Autodesk Inventor part; units mm, degrees
(part 10 of 18)
  ellipse E459 centre (-107.4, -28.6975) end of major axis (-107.4136, -28.887) minor radius 0.0836 (-107.3988, -28.8851) -> (-107.3155, -28.6702) ccw
  ellipse E460 centre (-107.3023, -23.1571) end of major axis (-107.2887, -22.9676) minor radius 0.0836 (-107.2177, -23.1298) -> (-107.2887, -22.9676) ccw
  ellipse E461 centre (-107.2657, -28.7071) end of major axis (-107.2793, -28.8966) minor radius 0.0836 (-107.2644, -28.8947) -> (-107.1812, -28.6798) ccw
  line L614 (-107.423, -22.958) -> (-107.2887, -22.9676)
  line L615 (-107.9988, -29.2688) -> (-108.1215, -29.26)
  line L616 (-108.1883, -29.2815) -> (-107.9671, -29.2974)
  ellipse E462 centre (-108.0103, -29.224) end of major axis (-108.2603, -29.2257) minor radius 0.0393 (-108.2342, -29.208) -> (-108.1215, -29.26) ccw
  ellipse E463 centre (-108.0103, -29.224) end of major axis (-107.6103, -29.2214) minor radius 0.0629 (-108.3653, -29.2553) -> (-108.1883, -29.2815) ccw
  line L617 (-87.4369, -24.724) -> (-87.3368, -24.7245)
  line L618 (-87.4451, -24.7415) -> (-87.4745, -24.7414)
  line L619 (-87.3116, -26.9591) -> (-87.5116, -24.9123)
  ellipse E464 centre (-87.2873, -23.1457) end of major axis (-87.3119, -22.9573) minor radius 0.0925 (-87.2875, -22.9605) -> (-87.3058, -22.9569) ccw
  ellipse E465 centre (-86.8717, -28.7468) end of major axis (-86.8472, -28.9352) minor radius 0.0925 (-86.8533, -28.9355) -> (-86.8472, -28.9352) ccw
  line L620 (-86.8467, -28.9351) -> (-86.8472, -28.9352)
  line L621 (-87.3058, -22.9569) -> (-87.3591, -22.9566)
  line L622 (-87.2928, -28.9157) -> (-86.9898, -28.9172)
  line L623 (-87.4747, -28.9323) -> (-87.092, -28.9343)
  line L624 (-86.8543, -28.9355) -> (-86.8533, -28.9355)
  ellipse E466 centre (-87.2185, -26.9596) end of major axis (-87.194, -27.148) minor radius 0.0925 (-87.3116, -26.9591) -> (-87.2495, -27.1225) ccw
  ellipse E467 centre (-87.4185, -24.9128) end of major axis (-87.443, -24.7244) minor radius 0.0925 (-87.4369, -24.724) -> (-87.5116, -24.9123) ccw
  line L625 (-106.3707, -22.9587) -> (-106.6076, -22.9637)
  line L626 (-106.9403, -28.9202) -> (-106.6983, -28.9152)
  line L627 (-106.8323, -28.9376) -> (-106.5774, -28.9323)
  line L628 (-106.6653, -24.7299) -> (-106.5258, -24.727)
  line L629 (-106.4991, -25.3055) -> (-106.6609, -26.9609)
  line L630 (-106.4907, -24.7459) -> (-106.5311, -24.7468)
  ellipse E468 centre (-106.5443, -24.9158) end of major axis (-106.5206, -24.7273) minor radius 0.0827 (-106.4591, -24.859) -> (-106.5258, -24.727) ccw
  ellipse E469 centre (-106.7442, -26.9627) end of major axis (-106.7205, -26.7741) minor radius 0.0827 (-106.7228, -27.13) -> (-106.6609, -26.9609) ccw
  ellipse E470 centre (-106.2503, -23.0086) end of major axis (-106.6484, -22.9697) minor radius 0.023 (-106.6076, -22.9637) -> (-106.6484, -22.9697) ccw
  line L631 (-106.6484, -22.9697) -> (-106.6497, -22.983)
  line L632 (-85.8205, -29.2346) -> (-85.9837, -29.2482)
  line L633 (-85.9794, -29.275) -> (-85.746, -29.2556)
  ellipse E471 centre (-85.8192, -29.047) end of major axis (-85.8707, -29.2299) minor radius 0.1628 (-85.8205, -29.2346) -> (-85.7328, -29.1988) ccw
  ellipse E472 centre (-85.7448, -29.0679) end of major axis (-85.7963, -29.2508) minor radius 0.1628 (-85.746, -29.2556) -> (-85.6862, -29.2378) ccw
  line L634 (-86.5987, -24.7323) -> (-86.4197, -24.7827)
  line L635 (-86.2178, -25.0275) -> (-86.2312, -27.0619)
  ellipse E473 centre (-86.9459, -24.7613) end of major axis (-86.5459, -24.764) minor radius 0.0629 (-86.5987, -24.7323) -> (-87.1444, -24.7054) ccw
  line L636 (-87.3451, -24.7222) -> (-87.1444, -24.7054)
  line L637 (-87.07, -24.7264) -> (-87.4891, -24.7614)
  ellipse E474 centre (-86.9459, -24.7613) end of major axis (-87.1959, -24.7597) minor radius 0.0393 (-86.7289, -24.7432) -> (-87.07, -24.7264) ccw
  line L638 (-86.5673, -24.7887) -> (-86.7289, -24.7432)
  line L639 (-87.1603, -27.115) -> (-87.2752, -27.1246)
  ellipse E475 centre (-86.9618, -27.1709) end of major axis (-87.3618, -27.1683) minor radius 0.0629 (-86.6549, -27.1325) -> (-87.1603, -27.115) ccw
  line L640 (-86.3614, -27.0727) -> (-86.3584, -26.6213)
  line L641 (-86.3511, -25.5132) -> (-86.348, -25.0384)
  ellipse E476 centre (-86.3121, -25.001) end of major axis (-86.3279, -24.8117) minor radius 0.0933 (-86.2178, -25.0275) -> (-86.2257, -24.9475) ccw
  ellipse E477 centre (-86.3255, -27.0353) end of major axis (-86.3413, -26.846) minor radius 0.0933 (-86.2481, -27.1626) -> (-86.2312, -27.0619) ccw
  ellipse E478 centre (-86.4423, -25.0119) end of major axis (-86.4265, -25.2012) minor radius 0.0933 (-86.348, -25.0384) -> (-86.3522, -24.9791) ccw
  ellipse E479 centre (-86.4557, -27.0462) end of major axis (-86.4399, -27.2355) minor radius 0.0933 (-86.3617, -27.0847) -> (-86.3614, -27.0727) ccw
  ellipse E480 centre (-86.4557, -27.0462) end of major axis (-86.4399, -27.2355) minor radius 0.0933 (-86.3709, -27.1501) -> (-86.3632, -27.1064) ccw
  line L642 (-86.6261, -28.8997) -> (-86.4729, -28.9429)
  line L643 (-86.7563, -28.9106) -> (-85.6745, -29.2152)
  line L644 (-87.1328, -22.9476) -> (-87.3502, -22.9658)
  ellipse E481 centre (-86.9734, -28.9287) end of major axis (-86.7234, -28.9304) minor radius 0.0393 (-86.7563, -28.9106) -> (-87.0903, -28.8932) ccw
  ellipse E482 centre (-86.9343, -23.0035) end of major axis (-87.3343, -23.0009) minor radius 0.0629 (-86.6073, -22.9694) -> (-87.1328, -22.9476) ccw
  ellipse E483 centre (-86.9734, -28.9287) end of major axis (-87.3734, -28.9261) minor radius 0.0629 (-86.6261, -28.8997) -> (-87.1678, -28.8725) ccw
  ellipse E484 centre (-85.6733, -29.0276) end of major axis (-85.6575, -29.2169) minor radius 0.0933 (-85.6745, -29.2152) -> (-85.6575, -29.2169) ccw
  line L645 (-85.6044, -29.2125) -> (-85.6575, -29.2169)
  ellipse E485 centre (-107.03, -29.085) end of major axis (-107.4723, -29.0961) minor radius 0.0741 (-107.1928, -29.02) -> (-107.2565, -29.0269) ccw
  ellipse E486 centre (-107.1797, -29.0466) end of major axis (-107.0298, -29.0428) minor radius 0.0251 (-107.2565, -29.0269) -> (-107.3177, -29.0401) ccw
  ellipse E487 centre (-107.5641, -29.2075) end of major axis (-107.714, -29.2112) minor radius 0.0251 (-107.7021, -29.201) -> (-107.714, -29.2103) ccw
  ellipse E488 centre (-107.5305, -29.2206) end of major axis (-107.6805, -29.2244) minor radius 0.0251 (-107.658, -29.2369) -> (-107.6551, -29.2376) ccw
  line L646 (-107.7021, -29.201) -> (-107.6522, -29.1801)
  line L647 (-107.5487, -29.1368) -> (-107.5155, -29.1229)
  line L648 (-107.3444, -29.0513) -> (-107.3177, -29.0401)
  line L649 (-106.0798, -29.1255) -> (-106.139, -29.1503)
  ellipse E489 centre (-106.8613, -29.1509) end of major axis (-106.2815, -29.1362) minor radius 0.0971 (-106.8801, -29.0542) -> (-107.3234, -29.1035) ccw
  ellipse E490 centre (-107.3553, -29.0674) end of major axis (-107.2055, -29.0598) minor radius 0.0268 (-107.3734, -29.0416) -> (-107.3848, -29.0425) ccw
  ellipse E491 centre (-107.3553, -29.0674) end of major axis (-107.2055, -29.0598) minor radius 0.0268 (-107.3195, -29.0396) -> (-107.3295, -29.0397) ccw
  ellipse E492 centre (-107.4395, -29.077) end of major axis (-107.2897, -29.0695) minor radius 0.0268 (-107.5122, -29.0571) -> (-107.5755, -29.0724) ccw
  ellipse E493 centre (-107.8512, -29.2569) end of major axis (-108.001, -29.2645) minor radius 0.0268 (-107.9872, -29.2523) -> (-107.9981, -29.2694) ccw
  ellipse E494 centre (-107.8202, -29.2705) end of major axis (-107.97, -29.278) minor radius 0.0268 (-107.9512, -29.2899) -> (-107.8831, -29.2979) ccw
  line L650 (-108.0017, -29.2505) -> (-108.001, -29.2645)
  ellipse E495 centre (-107.2977, -29.1159) end of major axis (-107.7396, -29.1382) minor radius 0.0791 (-107.3848, -29.0425) -> (-107.5122, -29.0571) ccw
  ellipse E496 centre (-107.5648, -29.2326) end of major axis (-108.0068, -29.2549) minor radius 0.0791 (-107.9981, -29.2694) -> (-107.9512, -29.2899) ccw
  line L651 (-107.9872, -29.2523) -> (-107.5755, -29.0724)
  line L652 (-107.6516, -29.3057) -> (-107.8831, -29.2979)
  ellipse E497 centre (-107.1421, -29.184) end of major axis (-107.7214, -29.2133) minor radius 0.1037 (-107.116, -29.079) -> (-107.6541, -29.2576) ccw
  ellipse E498 centre (-86.1558, -29.259) end of major axis (-86.3056, -29.2514) minor radius 0.0268 (-86.0793, -29.2858) -> (-86.018, -29.2763) ccw
  ellipse E499 centre (-86.1337, -29.2445) end of major axis (-85.9839, -29.2521) minor radius 0.0268 (-85.9845, -29.2543) -> (-86.0049, -29.2371) ccw
  ellipse E500 centre (-86.6351, -29.0687) end of major axis (-86.4852, -29.0763) minor radius 0.0268 (-86.5062, -29.0613) -> (-86.5762, -29.0469) ccw
  ellipse E501 centre (-86.722, -29.0605) end of major axis (-86.5722, -29.0681) minor radius 0.0268 (-86.79, -29.0332) -> (-86.7985, -29.0337) ccw
  line L653 (-85.9839, -29.2521) -> (-85.983, -29.2345)
  ellipse E502 centre (-86.4245, -29.2253) end of major axis (-85.9826, -29.2476) minor radius 0.0791 (-86.018, -29.2763) -> (-85.9845, -29.2543) ccw
  ellipse E503 centre (-86.7498, -29.1112) end of major axis (-87.1917, -29.0889) minor radius 0.0791 (-86.5762, -29.0469) -> (-86.628, -29.0411) ccw
  line L654 (-86.5062, -29.0613) -> (-86.0049, -29.2371)
  line L655 (-87.0813, -29.0499) -> (-87.0782, -29.0497)
  line L656 (-86.8628, -29.0374) -> (-86.7985, -29.0337)
  line L657 (-86.0793, -29.2858) -> (-86.3512, -29.3014)
  ellipse E504 centre (-86.8609, -29.184) end of major axis (-86.2817, -29.2133) minor radius 0.1037 (-86.349, -29.2576) -> (-86.8871, -29.079) ccw
  line L658 (-87.9857, -29.2296) -> (-87.8649, -29.2702)
  ellipse E505 centre (-88.4742, -29.4154) end of major axis (-87.8969, -29.3596) minor radius 0.1485 (-87.8979, -29.373) -> (-87.9795, -29.2938) ccw
  line L659 (-106.1382, -29.2698) -> (-106.0162, -29.2181)
  ellipse E506 centre (-105.5289, -29.4154) end of major axis (-106.1062, -29.3596) minor radius 0.1485 (-106.0236, -29.2938) -> (-106.1051, -29.373) ccw
  ellipse E507 centre (-106.8474, -29.0174) end of major axis (-106.6974, -29.0164) minor radius 0.0236 (-106.7807, -28.9958) -> (-106.8728, -28.9943) ccw
  ellipse E508 centre (-106.9325, -29.0224) end of major axis (-106.7825, -29.0214) minor radius 0.0236 (-107.0016, -29.0019) -> (-107.0669, -29.0128) ccw
  ellipse E509 centre (-106.7978, -29.0624) end of major axis (-107.2403, -29.0653) minor radius 0.0696 (-106.8728, -28.9943) -> (-107.0016, -29.0019) ccw
  line L660 (-107.1367, -29.0353) -> (-107.0669, -29.0128)
  line L661 (-106.0116, -29.1703) -> (-106.1386, -29.2113)
  line L662 (-106.7807, -28.9958) -> (-106, -29.0518)
  ellipse E510 centre (-106.6541, -29.1287) end of major axis (-106.0741, -29.1248) minor radius 0.0912 (-106.1389, -29.1672) -> (-107.1406, -29.0821) ccw
  ellipse E511 centre (-87.822, -29.0059) end of major axis (-87.9713, -29.0205) minor radius 0.0086 (-87.6911, -28.9974) -> (-87.6859, -28.9962) ccw
  ellipse E512 centre (-87.822, -29.0059) end of major axis (-87.9713, -29.0205) minor radius 0.0086 (-87.7484, -29.0063) -> (-87.7462, -29.006) ccw
  ellipse E513 centre (-87.7981, -28.9986) end of major axis (-87.6488, -28.984) minor radius 0.0086 (-87.6498, -28.9852) -> (-87.6682, -28.9817) ccw
  line L663 (-87.6488, -28.984) -> (-87.6515, -28.9565)
  ellipse E514 centre (-88.0872, -29.0248) end of major axis (-87.6468, -28.9818) minor radius 0.0254 (-87.6859, -28.9962) -> (-87.6498, -28.9852) ccw
  line L664 (-88.0608, -28.9797) -> (-87.6682, -28.9817)
  line L665 (-87.7484, -29.0063) -> (-88.0043, -29.0396)
  ellipse E515 centre (-88.5198, -29.06) end of major axis (-87.9425, -29.0036) minor radius 0.0333 (-88.0057, -29.0251) -> (-88.0631, -28.995) ccw
  line L666 (-106.3288, -28.9852) -> (-105.9427, -28.9771)
  line L667 (-105.9989, -29.0404) -> (-106.2318, -29.0111)
  ellipse E516 centre (-106.1948, -29.002) end of major axis (-106.3441, -28.9874) minor radius 0.0086 (-106.3288, -28.9852) -> (-106.3418, -28.9892) ccw
  ellipse E517 centre (-106.166, -29.0097) end of major axis (-106.3153, -28.9952) minor radius 0.0086 (-106.2982, -29.0009) -> (-106.2318, -29.0111) ccw
  line L668 (-106.3424, -28.9701) -> (-106.3441, -28.9874)
  ellipse E518 centre (-105.9081, -29.027) end of major axis (-106.3485, -28.984) minor radius 0.0254 (-106.3418, -28.9892) -> (-106.2982, -29.0009) ccw
  ellipse E519 centre (-105.4833, -29.06) end of major axis (-106.0606, -29.0036) minor radius 0.0333 (-105.94, -28.995) -> (-105.9974, -29.0251) ccw
  line L669 (-86.9808, -29.0089) -> (-86.8038, -29.0588)
  line L670 (-86.6763, -29.0947) -> (-86.6678, -29.0971)
  line L671 (-88.0027, -29.0555) -> (-87.2721, -28.9946)
  line L672 (-87.8645, -29.2069) -> (-87.9914, -29.1712)
  ellipse E520 centre (-87.111, -29.0198) end of major axis (-86.961, -29.0208) minor radius 0.0236 (-86.9808, -29.0089) -> (-87.0499, -28.9986) ccw
  ellipse E521 centre (-87.1977, -29.0155) end of major axis (-87.0477, -29.0165) minor radius 0.0236 (-87.1809, -28.9922) -> (-87.2721, -28.9946) ccw
  ellipse E522 centre (-87.2304, -29.061) end of major axis (-87.6729, -29.0581) minor radius 0.0696 (-87.0499, -28.9986) -> (-87.1809, -28.9922) ccw
  ellipse E523 centre (-87.349, -29.1287) end of major axis (-87.9289, -29.1248) minor radius 0.0912 (-86.8625, -29.0821) -> (-87.8642, -29.1672) ccw
  line L673 (-107.5835, -27.1193) -> (-107.6094, -27.1302)
  line L674 (-107.6509, -25.0431) -> (-107.636, -25.0368)
  line L675 (-107.5375, -27.1215) -> (-107.5621, -27.1318)
  line L676 (-107.5835, -27.1193) -> (-107.586, -27.0193)
  ellipse E524 centre (-107.4883, -26.9784) end of major axis (-107.4766, -26.7286) minor radius 0.0974 (-107.4945, -26.732) -> (-107.586, -27.0193) ccw
  line L677 (-107.4945, -26.732) -> (-107.1446, -26.5855)
  line L678 (-107.108, -26.4706) -> (-107.1381, -25.2781)
  line L679 (-107.1796, -25.1959) -> (-107.401, -25.2885)
  ellipse E525 centre (-107.5357, -25.0959) end of major axis (-107.524, -24.8462) minor radius 0.0974 (-107.6334, -25.1368) -> (-107.612, -25.2714) ccw
  line L680 (-107.6334, -25.1368) -> (-107.636, -25.0368)
  line L681 (-107.0921, -25.2802) -> (-107.062, -26.4728)
  line L682 (-107.59, -25.039) -> (-107.5874, -25.139)
  ellipse E526 centre (-107.4897, -25.0981) end of major axis (-107.5014, -25.3478) minor radius 0.0974 (-107.5874, -25.139) -> (-107.572, -25.254) ccw
  line L683 (-107.0986, -26.5877) -> (-107.4485, -26.7341)
  ellipse E527 centre (-107.4423, -26.9805) end of major axis (-107.4306, -26.7308) minor radius 0.0974 (-107.4485, -26.7341) -> (-107.54, -27.0214) ccw
  line L684 (-107.54, -27.0214) -> (-107.5375, -27.1215)
  line L685 (-107.636, -25.0368) -> (-107.59, -25.039)
  line L686 (-107.5375, -27.1215) -> (-107.5835, -27.1193)
  ellipse E528 centre (-107.1471, -26.487) end of major axis (-107.1518, -26.5869) minor radius 0.0389 (-107.1446, -26.5855) -> (-107.108, -26.4706) ccw
  ellipse E529 centre (-107.1772, -25.2944) end of major axis (-107.1725, -25.1945) minor radius 0.0389 (-107.1381, -25.2781) -> (-107.1796, -25.1959) ccw
  ellipse E530 centre (-107.1011, -26.4891) end of major axis (-107.1058, -26.589) minor radius 0.0389 (-107.0986, -26.5877) -> (-107.062, -26.4728) ccw
  ellipse E531 centre (-107.1312, -25.2966) end of major axis (-107.1265, -25.1967) minor radius 0.0389 (-107.0921, -25.2802) -> (-107.1265, -25.1967) ccw
  line L687 (-107.1725, -25.1945) -> (-107.1265, -25.1967)
  line L688 (-87.0844, -27.0597) -> (-87.1343, -27.0638)
  line L689 (-87.032, -24.9771) -> (-87.059, -24.9794)
  line L690 (-87.1278, -27.0733) -> (-87.0573, -27.0674)
  ellipse E532 centre (-86.8738, -26.7932) end of major axis (-86.8057, -26.5526) minor radius 0.2063 (-87.0767, -26.7545) -> (-87.0795, -26.8661) ccw
  ellipse E533 centre (-86.8339, -25.2093) end of major axis (-86.7658, -24.9688) minor radius 0.2063 (-87.0368, -25.1707) -> (-87.0396, -25.2823) ccw
  spline S43 degree 3 poles (-86.6514, -26.786) (-86.652, -26.7802) (-86.6533, -26.7686) (-86.6565, -26.7515) (-86.6607, -26.7348) (-86.6658, -26.7185) (-86.6719, -26.7028) (-86.6788, -26.6877) (-86.6865, -26.6732) (-86.6951, -26.6594) (-86.7044, -26.6464) (-86.7145, -26.6342) (-86.7252, -26.6228) (-86.7366, -26.6125) (-86.7487, -26.6031) (-86.7613, -26.5947) (-86.7744, -26.5875) (-86.7835, -26.5836) (-86.7881, -26.5817) knots 0 0 0 0 0.068015 0.135329 0.201939 0.267833 0.332993 0.397396 0.46102 0.523846 0.585863 0.647073 0.70749 0.767154 0.826125 0.884497 0.9424 1 1 1 1
  spline S44 degree 3 poles (-86.9219, -26.5886) (-86.9259, -26.5906) (-86.9339, -26.5947) (-86.9453, -26.6018) (-86.9564, -26.6096) (-86.9669, -26.6182) (-86.977, -26.6274) (-86.9866, -26.6373) (-86.9957, -26.6478) (-87.0042, -26.6588) (-87.0121, -26.6704) (-87.0195, -26.6824) (-87.0262, -26.6949) (-87.0323, -26.7077) (-87.0377, -26.7209) (-87.0424, -26.7344) (-87.0465, -26.7482) (-87.0485, -26.7575) (-87.0496, -26.7622) knots 0 0 0 0 0.060188 0.120572 0.181231 0.242221 0.303577 0.365317 0.427444 0.489947 0.552805 0.61599 0.67947 0.743206 0.807162 0.871301 0.93559 1 1 1 1
  spline S45 degree 3 poles (-87.0767, -26.7545) (-87.0755, -26.7499) (-87.0732, -26.7407) (-87.0683, -26.7272) (-87.0626, -26.714) (-87.0561, -26.7012) (-87.0487, -26.6887) (-87.0405, -26.6767) (-87.0316, -26.6651) (-87.0219, -26.654) (-87.0117, -26.6433) (-87.0008, -26.6332) (-86.9894, -26.6237) (-86.9774, -26.6147) (-86.965, -26.6063) (-86.9522, -26.5986) (-86.939, -26.5915) (-86.9299, -26.5874) (-86.9254, -26.5853) knots 0 0 0 0 0.060752 0.121577 0.182585 0.243852 0.305433 0.367353 0.42962 0.492223 0.555134 0.618315 0.681718 0.745286 0.808961 0.872679 0.936378 1 1 1 1
  spline S46 degree 3 poles (-86.8201, -26.5632) (-86.8129, -26.5635) (-86.7984, -26.5641) (-86.777, -26.5679) (-86.7562, -26.5737) (-86.7365, -26.5817) (-86.7182, -26.5915) (-86.7013, -26.6031) (-86.6858, -26.6163) (-86.6718, -26.6309) (-86.6591, -26.6468) (-86.6478, -26.6638) (-86.638, -26.6819) (-86.6295, -26.7008) (-86.6224, -26.7205) (-86.6166, -26.7407) (-86.6122, -26.7614) (-86.6104, -26.7754) (-86.6095, -26.7825) knots 0 0 0 0 0.06487 0.129748 0.194733 0.25818 0.320168 0.381236 0.441837 0.502335 0.563004 0.624034 0.685537 0.747559 0.810091 0.873076 0.936419 1 1 1 1
  spline S47 degree 3 poles (-86.6123, -26.8946) (-86.6135, -26.9008) (-86.616, -26.9132) (-86.6218, -26.9309) (-86.629, -26.9477) (-86.6377, -26.9634) (-86.6478, -26.978) (-86.6592, -26.9915) (-86.6718, -27.0037) (-86.6856, -27.0148) (-86.7005, -27.0246) (-86.7164, -27.0331) (-86.7333, -27.0403) (-86.7511, -27.0461) (-86.7697, -27.0505) (-86.789, -27.0534) (-86.8091, -27.055) (-86.8226, -27.0548) (-86.8295, -27.0546) knots 0 0 0 0 0.064651 0.127488 0.188893 0.249239 0.308882 0.368162 0.427398 0.486884 0.546892 0.60767 0.669446 0.732427 0.796802 0.862747 0.930428 1 1 1 1
  spline S48 degree 3 poles (-86.9339, -27.032) (-86.9386, -27.03) (-86.9479, -27.026) (-86.9614, -27.0191) (-86.9743, -27.0116) (-86.9867, -27.0035) (-86.9985, -26.9948) (-87.0096, -26.9855) (-87.0201, -26.9757) (-87.0299, -26.9653) (-87.039, -26.9544) (-87.0473, -26.9431) (-87.0548, -26.9313) (-87.0615, -26.919) (-87.0674, -26.9063) (-87.0724, -26.8933) (-87.0766, -26.8799) (-87.0786, -26.8707) (-87.0795, -26.8661) knots 0 0 0 0 0.066474 0.132184 0.19716 0.261439 0.325059 0.388062 0.450498 0.512425 0.573908 0.635026 0.695866 0.756532 0.81714 0.87782 0.938719 1 1 1 1
  spline S49 degree 3 poles (-87.0524, -26.8738) (-87.0518, -26.8773) (-87.0506, -26.8842) (-87.0481, -26.8943) (-87.0451, -26.9042) (-87.0416, -26.9139) (-87.0377, -26.9234) (-87.0319, -26.9357) (-87.0235, -26.9505) (-87.012, -26.9671) (-86.9989, -26.9827) (-86.9847, -26.9971) (-86.9743, -27.0057) (-86.9691, -27.01) knots 0 0 0 0 0.064451 0.128324 0.191723 0.254738 0.31745 0.379928 0.504372 0.628458 0.752389 0.876245 1 1 1 1
  spline S50 degree 3 poles (-86.7548, -27.0503) (-86.7513, -27.0487) (-86.7444, -27.0456) (-86.7346, -27.04) (-86.7253, -27.0336) (-86.7166, -27.0266) (-86.7084, -27.019) (-86.7008, -27.0107) (-86.6937, -27.0017) (-86.6872, -26.9922) (-86.6812, -26.9822) (-86.6757, -26.9716) (-86.6708, -26.9605) (-86.6664, -26.9489) (-86.6625, -26.9368) (-86.6592, -26.9243) (-86.6564, -26.9113) (-86.655, -26.9025) (-86.6542, -26.8981) knots 0 0 0 0 0.059947 0.119085 0.177737 0.236204 0.294771 0.353693 0.413202 0.473501 0.534763 0.597137 0.660745 0.725684 0.792031 0.859842 0.929157 1 1 1 1
  spline S51 degree 3 poles (-86.6115, -25.2022) (-86.6122, -25.1958) (-86.6136, -25.183) (-86.6174, -25.1643) (-86.6222, -25.146) (-86.6282, -25.1283) (-86.6353, -25.1113) (-86.6434, -25.095) (-86.6526, -25.0795) (-86.6626, -25.065) (-86.6736, -25.0514) (-86.6854, -25.0389) (-86.698, -25.0275) (-86.7114, -25.0173) (-86.7254, -25.0085) (-86.7401, -25.001) (-86.7553, -24.9949) (-86.7659, -24.9922) (-86.7712, -24.9908) knots 0 0 0 0 0.068478 0.136179 0.203098 0.269216 0.33451 0.398951 0.462515 0.525184 0.586956 0.647848 0.707903 0.767201 0.825862 0.884056 0.942007 1 1 1 1
  spline S52 degree 3 poles (-86.8981, -25.0135) (-86.9015, -25.0157) (-86.9085, -25.0201) (-86.9185, -25.0274) (-86.9281, -25.0353) (-86.9373, -25.0438) (-86.9461, -25.0529) (-86.9544, -25.0624) (-86.9623, -25.0724) (-86.9697, -25.0828) (-86.9767, -25.0937) (-86.9831, -25.1049) (-86.9889, -25.1165) (-86.9943, -25.1284) (-86.999, -25.1405) (-87.0032, -25.1529) (-87.0068, -25.1655) (-87.0087, -25.1741) (-87.0097, -25.1784) knots 0 0 0 0 0.06026 0.120787 0.181623 0.242797 0.30432 0.366196 0.428417 0.490967 0.553825 0.616963 0.680352 0.743961 0.807759 0.871715 0.935803 1 1 1 1
  spline S53 degree 3 poles (-87.0368, -25.1707) (-87.0357, -25.1664) (-87.0335, -25.1578) (-87.0291, -25.1453) (-87.024, -25.133) (-87.0181, -25.121) (-87.0115, -25.1094) (-87.0042, -25.0981) (-86.9962, -25.0871) (-86.9877, -25.0765) (-86.9785, -25.0664) (-86.9688, -25.0566) (-86.9586, -25.0474) (-86.9479, -25.0386) (-86.9368, -25.0303) (-86.9252, -25.0226) (-86.9134, -25.0154) (-86.9052, -25.011) (-86.9011, -25.0089) knots 0 0 0 0 0.060837 0.121734 0.182787 0.244069 0.305631 0.367501 0.429693 0.492205 0.555019 0.618108 0.681437 0.744961 0.808632 0.872398 0.936205 1 1 1 1
  spline S54 degree 3 poles (-86.8012, -24.98) (-86.7935, -24.9797) (-86.7782, -24.9789) (-86.7552, -24.9808) (-86.7326, -24.985) (-86.7108, -24.9918) (-86.6903, -25.0009) (-86.6714, -25.0121) (-86.6541, -25.0251) (-86.6384, -25.0398) (-86.6243, -25.0561) (-86.6118, -25.0737) (-86.6009, -25.0925) (-86.5915, -25.1123) (-86.5836, -25.133) (-86.5773, -25.1544) (-86.5725, -25.1763) (-86.5705, -25.1912) (-86.5695, -25.1986) knots 0 0 0 0 0.064914 0.129619 0.19438 0.258975 0.321768 0.383219 0.443897 0.504267 0.56469 0.625418 0.686613 0.748349 0.81063 0.873405 0.936573 1 1 1 1
  spline S55 degree 3 poles (-86.5724, -25.3107) (-86.5737, -25.3173) (-86.5763, -25.3304) (-86.5826, -25.3491) (-86.5904, -25.3666) (-86.5999, -25.383) (-86.6109, -25.3981) (-86.6234, -25.412) (-86.6372, -25.4245) (-86.6523, -25.4356) (-86.6686, -25.4453) (-86.6859, -25.4535) (-86.7044, -25.4603) (-86.7237, -25.4654) (-86.7439, -25.469) (-86.7649, -25.4709) (-86.7867, -25.4713) (-86.8013, -25.4701) (-86.8087, -25.4695) knots 0 0 0 0 0.064101 0.126323 0.187089 0.246808 0.305872 0.364653 0.423494 0.482714 0.542601 0.60342 0.665411 0.728789 0.793757 0.860499 0.92919 1 1 1 1
  spline S56 degree 3 poles (-86.9128, -25.4397) (-86.9168, -25.4376) (-86.925, -25.4334) (-86.9367, -25.4264) (-86.9479, -25.4189) (-86.9587, -25.4109) (-86.9689, -25.4024) (-86.9786, -25.3934) (-86.9877, -25.384) (-86.9962, -25.3742) (-87.004, -25.3639) (-87.0113, -25.3533) (-87.0178, -25.3423) (-87.0237, -25.331) (-87.0288, -25.3193) (-87.0332, -25.3072) (-87.0369, -25.2949) (-87.0387, -25.2865) (-87.0396, -25.2823) knots 0 0 0 0 0.065853 0.13104 0.19559 0.259537 0.322916 0.38577 0.448145 0.510097 0.571687 0.632987 0.694078 0.755051 0.81601 0.877068 0.938352 1 1 1 1
  spline S57 degree 3 poles (-87.0125, -25.29) (-87.0119, -25.2935) (-87.0106, -25.3003) (-87.0081, -25.3105) (-87.0052, -25.3204) (-87.0017, -25.3301) (-86.9978, -25.3396) (-86.992, -25.3519) (-86.9836, -25.3666) (-86.972, -25.3833) (-86.959, -25.3989) (-86.9448, -25.4133) (-86.9344, -25.4219) (-86.9292, -25.4262) knots 0 0 0 0 0.064451 0.128324 0.191723 0.254738 0.31745 0.379928 0.504372 0.628458 0.752389 0.876245 1 1 1 1
  spline S58 degree 3 poles (-86.7149, -25.4665) (-86.7114, -25.4649) (-86.7045, -25.4618) (-86.6947, -25.4561) (-86.6854, -25.4498) (-86.6767, -25.4428) (-86.6685, -25.4351) (-86.6609, -25.4268) (-86.6538, -25.4179) (-86.6473, -25.4084) (-86.6413, -25.3984) (-86.6358, -25.3878) (-86.6309, -25.3766) (-86.6265, -25.365) (-86.6226, -25.353) (-86.6193, -25.3404) (-86.6165, -25.3275) (-86.6151, -25.3187) (-86.6143, -25.3143) knots 0 0 0 0 0.059947 0.119085 0.177737 0.236204 0.294771 0.353693 0.413202 0.473501 0.534763 0.597137 0.660745 0.725684 0.792031 0.859842 0.929157 1 1 1 1
  ellipse E534 centre (-86.7431, -26.801) end of major axis (-86.7222, -27.0502) minor radius 0.1348 (-86.6123, -26.8946) -> (-86.6095, -26.7825) ccw
  ellipse E535 centre (-86.7851, -26.8046) end of major axis (-86.806, -26.5554) minor radius 0.1348 (-86.6542, -26.8981) -> (-86.6514, -26.786) ccw
  ellipse E536 centre (-86.7032, -25.2172) end of major axis (-86.6823, -25.4663) minor radius 0.1348 (-86.5724, -25.3107) -> (-86.5695, -25.1986) ccw
  ellipse E537 centre (-86.7452, -25.2207) end of major axis (-86.7661, -24.9716) minor radius 0.1348 (-86.6143, -25.3143) -> (-86.6115, -25.2022) ccw
  ellipse E538 centre (-86.8466, -26.8008) end of major axis (-86.9148, -27.0414) minor radius 0.2063 (-87.0496, -26.7622) -> (-87.0524, -26.8738) ccw
  ellipse E539 centre (-86.8067, -25.217) end of major axis (-86.8749, -25.4576) minor radius 0.2063 (-87.0097, -25.1784) -> (-87.0125, -25.29) ccw
  ellipse E540 centre (-86.9008, -27.1117) end of major axis (-86.6129, -27.1189) minor radius 0.0482 (-86.8837, -27.0639) -> (-87.0573, -27.0674) ccw
  ellipse E541 centre (-86.9008, -27.1117) end of major axis (-86.6129, -27.1189) minor radius 0.0482 (-86.6591, -27.0914) -> (-86.7868, -27.0702) ccw
  ellipse E542 centre (-86.9008, -27.1117) end of major axis (-87.2387, -27.1032) minor radius 0.0566 (-86.6172, -27.0879) -> (-86.8276, -27.0582) ccw
  ellipse E543 centre (-86.9008, -27.1117) end of major axis (-87.2387, -27.1032) minor radius 0.0566 (-86.956, -27.0545) -> (-87.0844, -27.0597) ccw
  ellipse E544 centre (-86.8483, -25.0292) end of major axis (-87.1862, -25.0206) minor radius 0.0566 (-86.5647, -25.0053) -> (-86.8279, -24.9732) ccw
  ellipse E545 centre (-86.8483, -25.0292) end of major axis (-87.1862, -25.0206) minor radius 0.0566 (-86.9657, -24.9732) -> (-87.032, -24.9771) ccw
  line L691 (-86.4051, -27.1479) -> (-86.6172, -27.0879)
  line L692 (-86.5647, -25.0053) -> (-86.5339, -25.014)
  line L693 (-86.4459, -25.039) -> (-86.3482, -25.0667)
  line L694 (-86.4689, -27.1452) -> (-86.6591, -27.0914)
  line L695 (-107.7479, -26.7469) -> (-107.4222, -26.6047)
  line L696 (-107.3853, -26.4881) -> (-107.4454, -25.2991)
  line L697 (-107.4923, -25.2191) -> (-107.867, -25.3828)
  ellipse E546 centre (-107.8794, -25.1371) end of major axis (-107.8879, -25.387) minor radius 0.1052 (-107.9777, -25.2426) -> (-107.867, -25.3828) ccw
  line L698 (-107.4001, -25.3006) -> (-107.34, -26.4896)
  line L699 (-107.3769, -26.6062) -> (-107.7032, -26.7487)
  line L700 (-107.9818, -25.0834) -> (-107.9788, -25.0835)
  ellipse E547 centre (-107.4272, -26.5064) end of major axis (-107.4306, -26.6063) minor radius 0.0421 (-107.4222, -26.6047) -> (-107.3853, -26.4881) ccw
  ellipse E548 centre (-107.4873, -25.3174) end of major axis (-107.4839, -25.2175) minor radius 0.0421 (-107.4454, -25.2991) -> (-107.4923, -25.2191) ccw
  ellipse E549 centre (-107.3819, -26.5079) end of major axis (-107.3852, -26.6079) minor radius 0.0421 (-107.3769, -26.6062) -> (-107.34, -26.4896) ccw
  ellipse E550 centre (-107.442, -25.3189) end of major axis (-107.4386, -25.219) minor radius 0.0421 (-107.4001, -25.3006) -> (-107.4386, -25.219) ccw
  line L701 (-107.4839, -25.2175) -> (-107.4386, -25.219)
  ellipse E551 centre (-87.4129, -25.3265) end of major axis (-87.4253, -25.2273) minor radius 0.0505 (-87.3991, -25.237) -> (-87.4241, -25.2272) ccw
  line L702 (-87.4241, -25.2272) -> (-87.4804, -25.2315)
  line L703 (-86.7771, -27.0917) -> (-86.933, -27.1007)
  line L704 (-86.8082, -27.1039) -> (-86.7464, -27.1004)
  ellipse E552 centre (-86.4901, -26.8273) end of major axis (-86.4074, -26.5914) minor radius 0.2103 (-86.7039, -26.88) -> (-86.702, -26.895) ccw
  ellipse E553 centre (-86.4901, -26.8273) end of major axis (-86.4074, -26.5914) minor radius 0.2103 (-86.6964, -26.7837) -> (-86.7021, -26.8121) ccw
  ellipse E554 centre (-86.4103, -25.2482) end of major axis (-86.3276, -25.0123) minor radius 0.2103 (-86.6166, -25.2046) -> (-86.6222, -25.3159) ccw
  spline S59 degree 3 poles (-86.3666, -26.6432) (-86.37, -26.6407) (-86.3766, -26.6357) (-86.3872, -26.6291) (-86.3981, -26.6232) (-86.4094, -26.6182) (-86.4211, -26.6141) (-86.4331, -26.611) (-86.4454, -26.6087) (-86.458, -26.6075) (-86.4709, -26.6073) (-86.484, -26.6082) (-86.4973, -26.6102) (-86.5107, -26.6133) (-86.5238, -26.6174) (-86.5367, -26.6225) (-86.5491, -26.6285) (-86.5571, -26.6331) (-86.5611, -26.6355) knots 0 0 0 0 0.060272 0.120085 0.179563 0.238863 0.298168 0.35769 0.417672 0.478383 0.540118 0.603193 0.66794 0.734231 0.800525 0.866826 0.93328 1 1 1 1
  spline S60 degree 3 poles (-86.6561, -26.7482) (-86.6576, -26.7518) (-86.6606, -26.759) (-86.6646, -26.77) (-86.6681, -26.7812) (-86.67, -26.7888) (-86.6709, -26.7926) knots 0 0 0 0 0.249453 0.499322 0.749525 1 1 1 1
  spline S61 degree 3 poles (-86.6964, -26.7837) (-86.6955, -26.7806) (-86.6937, -26.7743) (-86.6905, -26.7652) (-86.6868, -26.7561) (-86.6827, -26.7472) (-86.6782, -26.7385) (-86.6733, -26.73) (-86.6681, -26.7216) (-86.6643, -26.7163) (-86.6624, -26.7136) knots 0 0 0 0 0.124037 0.24816 0.37249 0.497125 0.622143 0.747603 0.873547 1 1 1 1
  spline S62 degree 3 poles (-86.5851, -26.6424) (-86.5806, -26.6397) (-86.5716, -26.6343) (-86.5576, -26.6271) (-86.5433, -26.6206) (-86.5287, -26.615) (-86.5138, -26.6102) (-86.4988, -26.6063) (-86.4836, -26.6033) (-86.4683, -26.6012) (-86.453, -26.6002) (-86.4378, -26.6001) (-86.4226, -26.601) (-86.4076, -26.6031) (-86.3928, -26.6062) (-86.3783, -26.6106) (-86.3643, -26.6159) (-86.3555, -26.6203) (-86.3511, -26.6224) knots 0 0 0 0 0.06406 0.128101 0.192047 0.25583 0.319386 0.382665 0.44563 0.508261 0.570562 0.63256 0.694313 0.755909 0.817476 0.879176 0.940214 1 1 1 1
  spline S63 degree 3 poles (-86.3634, -27.0803) (-86.3678, -27.0816) (-86.3768, -27.0843) (-86.3906, -27.0873) (-86.4048, -27.0895) (-86.4194, -27.0909) (-86.4344, -27.0914) (-86.4498, -27.091) (-86.4655, -27.0897) (-86.4816, -27.0876) (-86.4978, -27.0845) (-86.5142, -27.0806) (-86.5304, -27.0757) (-86.5462, -27.0701) (-86.5615, -27.0636) (-86.5763, -27.0564) (-86.5904, -27.0485) (-86.5994, -27.0426) (-86.6039, -27.0397) knots 0 0 0 0 0.054976 0.110963 0.168068 0.226392 0.286031 0.347076 0.409614 0.473728 0.539499 0.606943 0.674365 0.741 0.806864 0.871974 0.936347 1 1 1 1
  spline S64 degree 3 poles (-86.6726, -26.9699) (-86.6744, -26.9671) (-86.678, -26.9613) (-86.6828, -26.9524) (-86.6872, -26.9433) (-86.6911, -26.934) (-86.6946, -26.9245) (-86.6976, -26.9148) (-86.7001, -26.905) (-86.7014, -26.8983) (-86.702, -26.895) knots 0 0 0 0 0.125299 0.25024 0.374942 0.499537 0.624172 0.749009 0.874221 1 1 1 1
  spline S65 degree 3 poles (-86.6765, -26.9039) (-86.6762, -26.9059) (-86.6757, -26.9098) (-86.6746, -26.9155) (-86.6734, -26.9212) (-86.672, -26.9268) (-86.6704, -26.9324) (-86.6687, -26.9379) (-86.6668, -26.9434) (-86.6655, -26.9469) (-86.6648, -26.9487) knots 0 0 0 0 0.12683 0.253009 0.378607 0.503687 0.628312 0.752538 0.876418 1 1 1 1
  spline S66 degree 3 poles (-86.3824, -27.0888) (-86.3806, -27.0881) (-86.3772, -27.0867) (-86.3721, -27.0843) (-86.3671, -27.0817) (-86.364, -27.0798) (-86.3624, -27.0789) knots 0 0 0 0 0.252829 0.503515 0.752446 1 1 1 1
  spline S67 degree 3 poles (-86.3516, -25.0324) (-86.3547, -25.0317) (-86.361, -25.0304) (-86.3706, -25.0291) (-86.3803, -25.0284) (-86.3902, -25.0283) (-86.4003, -25.0288) (-86.4105, -25.03) (-86.4208, -25.0318) (-86.431, -25.0343) (-86.4412, -25.0374) (-86.4512, -25.0411) (-86.4609, -25.0453) (-86.4704, -25.0501) (-86.4797, -25.0553) (-86.4887, -25.0611) (-86.4975, -25.0674) (-86.5031, -25.0719) (-86.5059, -25.0741) knots 0 0 0 0 0.057782 0.11603 0.174905 0.234579 0.295234 0.357058 0.420245 0.484367 0.548389 0.61239 0.67646 0.740675 0.805095 0.869768 0.934728 1 1 1 1
  spline S68 degree 3 poles (-86.6166, -25.2046) (-86.6163, -25.2035) (-86.6157, -25.2013) (-86.6147, -25.1979) (-86.6136, -25.1946) (-86.6129, -25.1925) (-86.6125, -25.1914) knots 0 0 0 0 0.249966 0.499931 0.749931 1 1 1 1
  spline S69 degree 3 poles (-86.5301, -25.0806) (-86.5235, -25.0757) (-86.5102, -25.0659) (-86.4887, -25.0533) (-86.4664, -25.0425) (-86.4432, -25.0337) (-86.4195, -25.0271) (-86.3995, -25.0234) (-86.3834, -25.0217) (-86.3713, -25.021) (-86.3593, -25.021) (-86.3513, -25.0215) (-86.3473, -25.0217) knots 0 0 0 0 0.126262 0.252787 0.379198 0.50514 0.630313 0.754513 0.81624 0.877714 0.938955 1 1 1 1
  spline S70 degree 3 poles (-86.3498, -25.512) (-86.3582, -25.512) (-86.371, -25.512) (-86.3881, -25.5103) (-86.4013, -25.5085) (-86.4146, -25.5061) (-86.4326, -25.502) (-86.4548, -25.4955) (-86.4803, -25.4854) (-86.5043, -25.4733) (-86.523, -25.4615) (-86.5371, -25.4512) (-86.5438, -25.4457) (-86.5471, -25.443) knots 0 0 0 0 0.118368 0.179357 0.241611 0.305185 0.370129 0.500874 0.629162 0.755042 0.878604 0.939568 1 1 1 1
  spline S71 degree 3 poles (-86.6179, -25.335) (-86.6183, -25.3334) (-86.6192, -25.3303) (-86.6203, -25.3255) (-86.6213, -25.3207) (-86.6219, -25.3175) (-86.6222, -25.3159) knots 0 0 0 0 0.249221 0.498902 0.749131 1 1 1 1
  ellipse E555 centre (-86.4646, -26.8363) end of major axis (-86.5473, -27.0722) minor radius 0.2103 (-86.6709, -26.7926) -> (-86.6775, -26.8276) ccw
  ellipse E556 centre (-86.4646, -26.8363) end of major axis (-86.5473, -27.0722) minor radius 0.2103 (-86.679, -26.8825) -> (-86.6765, -26.9039) ccw
  ellipse E557 centre (-86.5394, -27.1484) end of major axis (-86.2518, -27.1629) minor radius 0.0515 (-86.6453, -27.0953) -> (-86.6848, -27.0968) ccw
  ellipse E558 centre (-86.5394, -27.1484) end of major axis (-86.2518, -27.1629) minor radius 0.0515 (-86.3643, -27.1161) -> (-86.5779, -27.0954) ccw
  ellipse E559 centre (-86.5394, -27.1484) end of major axis (-86.877, -27.1313) minor radius 0.0604 (-86.3586, -27.1062) -> (-86.6074, -27.0858) ccw
  ellipse E560 centre (-86.5394, -27.1484) end of major axis (-86.877, -27.1313) minor radius 0.0604 (-86.6784, -27.0865) -> (-86.7096, -27.0878) ccw
  ellipse E561 centre (-86.4344, -25.0721) end of major axis (-86.772, -25.055) minor radius 0.0604 (-86.3484, -25.0178) -> (-86.5497, -25.0096) ccw
  line L705 (-85.361, -27.0916) -> (-85.0567, -27.1982)
  line L706 (-85.0008, -27.1179) -> (-84.9406, -25.9289)
  line L707 (-84.9867, -25.8127) -> (-85.291, -25.706)
  line L708 (-85.0997, -27.2007) -> (-85.3619, -27.1088)
  ellipse E562 centre (-85.0518, -27.1) end of major axis (-85.046, -27.1998) minor radius 0.051 (-85.0567, -27.1982) -> (-85.0008, -27.1179) ccw
  ellipse E563 centre (-84.9916, -25.911) end of major axis (-84.9974, -25.8111) minor radius 0.051 (-84.9406, -25.9289) -> (-84.9867, -25.8127) ccw
  ellipse E564 centre (-85.0947, -27.1024) end of major axis (-85.089, -27.2023) minor radius 0.051 (-85.0997, -27.2007) -> (-85.089, -27.2023) ccw
  line L709 (-85.046, -27.1998) -> (-85.089, -27.2023)
  line L710 (-107.288, -27.0838) -> (-107.3343, -27.0988)
  line L711 (-107.468, -25.0508) -> (-107.3018, -24.9971)
  line L712 (-107.2432, -27.087) -> (-107.2865, -27.101)
  line L713 (-107.288, -27.0838) -> (-107.2887, -26.9836)
  ellipse E565 centre (-107.1775, -26.9476) end of major axis (-107.1596, -26.6983) minor radius 0.1101 (-107.1791, -26.7008) -> (-107.2887, -26.9836) ccw
  line L714 (-107.1791, -26.7008) -> (-106.7811, -26.5722)
  line L715 (-106.7373, -26.4591) -> (-106.7452, -25.2642)
  line L716 (-106.7903, -25.1798) -> (-107.0922, -25.2773)
  ellipse E566 centre (-107.1899, -25.0614) end of major axis (-107.172, -24.8121) minor radius 0.1101 (-107.3011, -25.0974) -> (-107.2783, -25.2372) ccw
  line L717 (-107.3011, -25.0974) -> (-107.3018, -24.9971)
  line L718 (-106.7004, -25.2674) -> (-106.6925, -26.4623)
  line L719 (-107.257, -25.0003) -> (-107.2563, -25.1006)
  ellipse E567 centre (-107.1451, -25.0646) end of major axis (-107.163, -25.314) minor radius 0.1101 (-107.2563, -25.1006) -> (-107.24, -25.2212) ccw
  line L720 (-106.7364, -26.5754) -> (-107.1343, -26.704)
  ellipse E568 centre (-107.1327, -26.9508) end of major axis (-107.1148, -26.7015) minor radius 0.1101 (-107.1343, -26.704) -> (-107.2439, -26.9868) ccw
  line L721 (-107.2439, -26.9868) -> (-107.2432, -27.087)
  line L722 (-107.3018, -24.9971) -> (-107.257, -25.0003)
  line L723 (-107.2432, -27.087) -> (-107.288, -27.0838)
  ellipse E569 centre (-106.7818, -26.4734) end of major axis (-106.7889, -26.5732) minor radius 0.044 (-106.7811, -26.5722) -> (-106.7373, -26.4591) ccw
  ellipse E570 centre (-106.7897, -25.2785) end of major axis (-106.7825, -25.1788) minor radius 0.044 (-106.7452, -25.2642) -> (-106.7903, -25.1798) ccw
  ellipse E571 centre (-106.737, -26.4767) end of major axis (-106.7442, -26.5764) minor radius 0.044 (-106.7364, -26.5754) -> (-106.6925, -26.4623) ccw
  ellipse E572 centre (-106.7449, -25.2817) end of major axis (-106.7377, -25.182) minor radius 0.044 (-106.7004, -25.2674) -> (-106.7377, -25.182) ccw
  line L724 (-106.7825, -25.1788) -> (-106.7377, -25.182)
  line L725 (-87.264, -27.0459) -> (-87.2919, -27.0482)
  line L726 (-87.2503, -24.9592) -> (-87.4582, -24.9766)
  line L727 (-87.2886, -27.057) -> (-87.2392, -27.0529)
  ellipse E573 centre (-87.051, -26.7784) end of major axis (-86.9832, -26.5378) minor radius 0.2142 (-87.262, -26.7401) -> (-87.2627, -26.852) ccw
  ellipse E574 centre (-87.0405, -25.1914) end of major axis (-86.9728, -24.9508) minor radius 0.2142 (-87.2515, -25.1532) -> (-87.2523, -25.265) ccw
  spline S72 degree 3 poles (-86.8442, -26.7663) (-86.8461, -26.7526) (-86.8499, -26.7258) (-86.8622, -26.6876) (-86.8789, -26.6526) (-86.9001, -26.6216) (-86.9251, -26.5953) (-86.9537, -26.5745) (-86.9802, -26.5625) (-87.0025, -26.5566) (-87.0198, -26.5541) (-87.0377, -26.5536) (-87.056, -26.5551) (-87.0746, -26.5588) (-87.093, -26.5646) (-87.1109, -26.5724) (-87.1337, -26.5852) (-87.1601, -26.6054) (-87.1874, -26.635) (-87.2098, -26.6692) (-87.2274, -26.7067) (-87.2339, -26.7336) (-87.2372, -26.7471) knots 0 0 0 0 0.067054 0.132171 0.195214 0.256087 0.314845 0.371833 0.427831 0.455897 0.484265 0.513193 0.542966 0.573892 0.605563 0.637232 0.669027 0.733247 0.798614 0.865047 0.932273 1 1 1 1
  spline S73 degree 3 poles (-87.262, -26.7401) (-87.2602, -26.7333) (-87.2567, -26.7197) (-87.246, -26.6935) (-87.2279, -26.6624) (-87.1997, -26.6292) (-87.1663, -26.6005) (-87.1288, -26.577) (-87.0884, -26.5595) (-87.0462, -26.5486) (-87.0103, -26.5458) (-86.982, -26.5478) (-86.9612, -26.5514) (-86.9411, -26.5572) (-86.9222, -26.5651) (-86.9047, -26.5748) (-86.8832, -26.59) (-86.8597, -26.613) (-86.8369, -26.6456) (-86.8196, -26.6821) (-86.8071, -26.7214) (-86.8029, -26.7488) (-86.8008, -26.7626) knots 0 0 0 0 0.031337 0.062781 0.126297 0.190936 0.256459 0.32232 0.387875 0.452577 0.516183 0.547678 0.57907 0.610325 0.640706 0.670386 0.69965 0.757762 0.816478 0.876441 0.937726 1 1 1 1
  spline S74 degree 3 poles (-86.8016, -26.8749) (-86.8039, -26.8874) (-86.8085, -26.9117) (-86.8234, -26.945) (-86.8435, -26.974) (-86.8687, -26.9982) (-86.8985, -27.0172) (-86.9324, -27.0307) (-86.9698, -27.0384) (-87.0103, -27.0399) (-87.0529, -27.0351) (-87.0957, -27.0243) (-87.1363, -27.0072) (-87.173, -26.9848) (-87.2049, -26.9576) (-87.227, -26.9312) (-87.2414, -26.9083) (-87.2504, -26.8903) (-87.2578, -26.8715) (-87.2611, -26.8585) (-87.2627, -26.852) knots 0 0 0 0 0.060227 0.117303 0.172542 0.227241 0.282631 0.339845 0.399897 0.463695 0.532058 0.603464 0.673189 0.741116 0.807351 0.872143 0.90418 0.93608 0.967968 1 1 1 1
  spline S75 degree 3 poles (-87.2379, -26.859) (-87.2373, -26.8623) (-87.2359, -26.8688) (-87.2333, -26.8785) (-87.2303, -26.888) (-87.2257, -26.9004) (-87.2188, -26.9153) (-87.209, -26.9323) (-87.1977, -26.9484) (-87.1852, -26.9635) (-87.1715, -26.9775) (-87.1616, -26.9859) (-87.1566, -26.9901) knots 0 0 0 0 0.06406 0.127639 0.190828 0.253706 0.37877 0.503307 0.627605 0.751814 0.875967 1 1 1 1
  spline S76 degree 3 poles (-86.9431, -27.0356) (-86.9396, -27.0341) (-86.9325, -27.031) (-86.9226, -27.0254) (-86.9132, -27.019) (-86.9045, -27.0119) (-86.8963, -27.004) (-86.8888, -26.9955) (-86.8819, -26.9863) (-86.8755, -26.9765) (-86.8697, -26.966) (-86.8645, -26.955) (-86.8599, -26.9435) (-86.8558, -26.9314) (-86.8523, -26.9189) (-86.8493, -26.9058) (-86.8468, -26.8924) (-86.8456, -26.8832) (-86.845, -26.8786) knots 0 0 0 0 0.059633 0.118254 0.176262 0.234034 0.291919 0.350232 0.409251 0.469215 0.530325 0.592744 0.656603 0.721998 0.789001 0.857656 0.927988 1 1 1 1
  spline S77 degree 3 poles (-86.8338, -25.1793) (-86.8357, -25.1657) (-86.8394, -25.1388) (-86.8518, -25.1007) (-86.8685, -25.0657) (-86.8896, -25.0346) (-86.9147, -25.0083) (-86.9433, -24.9876) (-86.9698, -24.9756) (-86.9921, -24.9697) (-87.0094, -24.9671) (-87.0272, -24.9666) (-87.0455, -24.9681) (-87.0641, -24.9719) (-87.0825, -24.9777) (-87.1004, -24.9854) (-87.1233, -24.9982) (-87.1496, -25.0184) (-87.177, -25.048) (-87.1994, -25.0822) (-87.2169, -25.1198) (-87.2235, -25.1466) (-87.2267, -25.1601) knots 0 0 0 0 0.067054 0.132171 0.195214 0.256087 0.314845 0.371833 0.427831 0.455897 0.484265 0.513193 0.542966 0.573892 0.605563 0.637232 0.669027 0.733247 0.798614 0.865047 0.932273 1 1 1 1
  spline S78 degree 3 poles (-87.2515, -25.1532) (-87.2498, -25.1464) (-87.2463, -25.1327) (-87.2356, -25.1065) (-87.2175, -25.0754) (-87.1893, -25.0422) (-87.1559, -25.0135) (-87.1184, -24.99) (-87.0779, -24.9725) (-87.0357, -24.9616) (-86.9998, -24.9588) (-86.9715, -24.9608) (-86.9507, -24.9644) (-86.9307, -24.9703) (-86.9118, -24.9781) (-86.8942, -24.9878) (-86.8728, -25.003) (-86.8492, -25.026) (-86.8264, -25.0586) (-86.8091, -25.0952) (-86.7966, -25.1345) (-86.7925, -25.1619) (-86.7904, -25.1757) knots 0 0 0 0 0.031337 0.062781 0.126297 0.190936 0.256459 0.32232 0.387875 0.452577 0.516183 0.547678 0.57907 0.610325 0.640706 0.670386 0.69965 0.757762 0.816478 0.876441 0.937726 1 1 1 1
  spline S79 degree 3 poles (-86.7911, -25.288) (-86.7935, -25.3004) (-86.7981, -25.3247) (-86.813, -25.3581) (-86.833, -25.3871) (-86.8583, -25.4112) (-86.8881, -25.4302) (-86.9219, -25.4437) (-86.9594, -25.4514) (-86.9998, -25.4529) (-87.0425, -25.4481) (-87.0852, -25.4373) (-87.1259, -25.4203) (-87.1625, -25.3979) (-87.1945, -25.3707) (-87.2166, -25.3443) (-87.231, -25.3213) (-87.24, -25.3033) (-87.2474, -25.2846) (-87.2506, -25.2715) (-87.2523, -25.265) knots 0 0 0 0 0.060227 0.117303 0.172542 0.227241 0.282631 0.339845 0.399897 0.463695 0.532058 0.603464 0.673189 0.741116 0.807351 0.872143 0.90418 0.93608 0.967968 1 1 1 1
  spline S80 degree 3 poles (-87.2275, -25.272) (-87.2268, -25.2753) (-87.2255, -25.2819) (-87.2229, -25.2916) (-87.2198, -25.301) (-87.2152, -25.3134) (-87.2083, -25.3283) (-87.1985, -25.3454) (-87.1873, -25.3614) (-87.1747, -25.3765) (-87.1611, -25.3905) (-87.1511, -25.3989) (-87.1461, -25.4032) knots 0 0 0 0 0.06406 0.127639 0.190828 0.253706 0.37877 0.503307 0.627605 0.751814 0.875967 1 1 1 1
  spline S81 degree 3 poles (-86.9327, -25.4486) (-86.9291, -25.4471) (-86.9221, -25.444) (-86.9121, -25.4384) (-86.9028, -25.432) (-86.894, -25.4249) (-86.8859, -25.417) (-86.8783, -25.4085) (-86.8714, -25.3993) (-86.865, -25.3895) (-86.8593, -25.3791) (-86.8541, -25.3681) (-86.8494, -25.3565) (-86.8453, -25.3445) (-86.8418, -25.3319) (-86.8388, -25.3189) (-86.8363, -25.3054) (-86.8351, -25.2962) (-86.8345, -25.2916) knots 0 0 0 0 0.059633 0.118254 0.176262 0.234034 0.291919 0.350232 0.409251 0.469215 0.530325 0.592744 0.656603 0.721998 0.789001 0.857656 0.927988 1 1 1 1
  ellipse E575 centre (-86.922, -26.7848) end of major axis (-86.9012, -27.0339) minor radius 0.1227 (-86.8016, -26.8749) -> (-86.8008, -26.7626) ccw
  ellipse E576 centre (-86.9654, -26.7884) end of major axis (-86.9862, -26.5393) minor radius 0.1227 (-86.845, -26.8786) -> (-86.8442, -26.7663) ccw
  ellipse E577 centre (-86.9116, -25.1978) end of major axis (-86.8908, -25.4469) minor radius 0.1227 (-86.7911, -25.288) -> (-86.7904, -25.1757) ccw
  ellipse E578 centre (-86.955, -25.2014) end of major axis (-86.9758, -24.9523) minor radius 0.1227 (-86.8345, -25.2916) -> (-86.8338, -25.1793) ccw
  ellipse E579 centre (-87.0262, -26.7854) end of major axis (-87.0939, -27.026) minor radius 0.2142 (-87.2372, -26.7471) -> (-87.2379, -26.859) ccw
  ellipse E580 centre (-87.0157, -25.1984) end of major axis (-87.0835, -25.4391) minor radius 0.2142 (-87.2267, -25.1601) -> (-87.2275, -25.272) ccw
  ellipse E581 centre (-87.0963, -27.0931) end of major axis (-86.8083, -27.095) minor radius 0.0453 (-86.8463, -27.0723) -> (-87.2392, -27.0529) ccw
  ellipse E582 centre (-87.0963, -27.0931) end of major axis (-87.4343, -27.0909) minor radius 0.0531 (-86.8029, -27.0686) -> (-87.264, -27.0459) ccw
  ellipse E583 centre (-87.0825, -25.0065) end of major axis (-87.4205, -25.0042) minor radius 0.0531 (-86.7891, -24.982) -> (-87.2503, -24.9592) ccw
  line L728 (-86.6436, -27.1135) -> (-86.8029, -27.0686)
  line L729 (-86.7891, -24.982) -> (-86.7725, -24.9867)
  line L730 (-86.7568, -24.9911) -> (-86.7439, -24.9947)
  line L731 (-86.6857, -27.1175) -> (-86.8463, -27.0723)
  line L732 (-107.5622, -25.0144) -> (-107.4557, -25.0194)
  ellipse E584 centre (-86.5423, -24.6872) end of major axis (-86.6268, -24.9855) minor radius 0.2558 (-86.55, -24.9928) -> (-86.5362, -24.9912) ccw
  line L733 (-86.5362, -24.9912) -> (-86.4689, -25.0102)
  line L734 (-86.5996, -24.9969) -> (-86.55, -24.9928)
  arc A8 (-108.8228, -25.1565) -> (-108.7216, -25.2665) centre (-108.5508, -25.0078) ccw
  ellipse E585 centre (-86.5473, -25.1031) end of major axis (-86.1053, -25.1255) minor radius 0.0791 (-86.348, -25.0422) -> (-86.3601, -25.0405) ccw
  arc A9 (-85.2685, -25.2613) -> (-85.1432, -25.1389) centre (-85.4136, -24.9873) ccw
  ellipse E586 centre (-107.2716, -24.667) end of major axis (-107.1763, -24.962) minor radius 0.274 (-107.2844, -24.9716) -> (-107.2696, -24.9731) ccw
  line L735 (-107.2998, -24.9766) -> (-107.2844, -24.9716)
  line L736 (-107.2696, -24.9731) -> (-107.1301, -24.9831)
  ellipse E587 centre (-87.3447, -24.6338) end of major axis (-87.319, -24.9428) minor radius 0.1522 (-87.3554, -24.937) -> (-87.3468, -24.94) ccw
  line L737 (-87.4552, -24.9454) -> (-87.3554, -24.937)
  ellipse E588 centre (-86.7811, -24.6615) end of major axis (-86.8651, -24.9599) minor radius 0.2656 (-86.7831, -24.9676) -> (-86.7687, -24.966) ccw
  line L738 (-86.7687, -24.966) -> (-86.7189, -24.98)
  line L739 (-86.8346, -24.9719) -> (-86.7831, -24.9676)
  line L740 (-87.3468, -24.94) -> (-87.294, -24.9548)
  ellipse E589 centre (-87.204, -25.0329) end of major axis (-86.7615, -25.0358) minor radius 0.0696 (-86.9838, -24.974) -> (-87.0099, -24.9716) ccw
  arc A10 (-107.3618, -27.0975) -> (-107.4959, -27.1212) centre (-107.3762, -27.4071) ccw
  line L741 (-107.4959, -27.1212) -> (-107.5417, -27.1403)
  line L742 (-107.036, -27.1127) -> (-107.3618, -27.0975)
  arc A11 (-107.7683, -27.1484) -> (-107.7835, -27.1546) centre (-107.6594, -27.4387) ccw
  arc A12 (-107.6489, -27.1289) -> (-107.7404, -27.1394) centre (-107.6594, -27.4387) ccw
  line L743 (-107.7835, -27.1546) -> (-107.8737, -27.194)
  line L744 (-107.5243, -27.1331) -> (-107.6489, -27.1289)
  arc A13 (-106.4029, -32.4979) -> (-106.4009, -32.4972) centre (-106.8054, -31.3674) ccw
  line L745 (-87.8189, -31.562) -> (-87.72, -32.5058)
  line L746 (-106.1842, -31.562) -> (-106.2831, -32.5058)
  arc A14 (-87.6022, -32.4972) -> (-87.6002, -32.4979) centre (-87.1977, -31.3674) ccw
  arc A15 (-90.5985, -35.3382) -> (-90.4829, -35.3126) centre (-90.7995, -34.1551) ccw
  line L747 (-90.296, -34.0468) -> (-90.2831, -34.1051)
  arc A16 (-103.5202, -35.3126) -> (-103.4046, -35.3382) centre (-103.2036, -34.1551) ccw
  line L748 (-103.7071, -34.0468) -> (-103.7199, -34.1051)
  arc A17 (-107.2677, -34.3213) -> (-106.7778, -34.3555) centre (-106.9408, -33.1666) ccw
  line L749 (-108.0363, -21.6967) -> (-108.0269, -21.8841)
  line L750 (-107.9752, -22.9062) -> (-107.968, -23.049)
  line L751 (-107.6573, -29.1932) -> (-107.5403, -31.5077)
  line L752 (-107.4859, -32.5836) -> (-107.4515, -33.2651)
  arc A18 (-104.3538, -35.2232) -> (-104.2354, -35.2295) centre (-104.2317, -34.0295) ccw
  line L753 (-103.7167, -34.0438) -> (-103.7199, -34.1051)
  line L754 (-104.7061, -33.2435) -> (-104.7563, -34.1999)
  line L755 (-91.4937, -33.0969) -> (-91.4774, -33.1737)
  arc A19 (-88.1095, -35.5428) -> (-87.8105, -35.509) centre (-88.0934, -34.3429) ccw
  line L756 (-87.667, -33.5285) -> (-87.5609, -34.4691)
  line L757 (-88.6914, -33.6357) -> (-88.5844, -34.5846)
  arc A20 (-106.1926, -35.509) -> (-105.8936, -35.5428) centre (-105.9097, -34.3429) ccw
  line L758 (-105.3117, -33.6357) -> (-105.4187, -34.5846)
  line L759 (-106.3361, -33.5285) -> (-106.4422, -34.4691)
  line L760 (-102.5094, -33.0969) -> (-102.5257, -33.1737)
  arc A21 (-89.7677, -35.2295) -> (-89.6493, -35.2232) centre (-89.7714, -34.0295) ccw
  line L761 (-89.297, -33.2435) -> (-89.2467, -34.1999)
  line L762 (-90.2864, -34.0438) -> (-90.2831, -34.1051)
  arc A22 (-87.2253, -34.3555) -> (-86.7354, -34.3213) centre (-87.0623, -33.1666) ccw
  line L763 (-85.9668, -21.6967) -> (-85.9762, -21.8841)
  line L764 (-86.0279, -22.9062) -> (-86.0335, -23.0165)
  line L765 (-86.3442, -29.1624) -> (-86.4628, -31.5077)